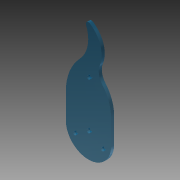
# Autodesk Inventor part: tail_bottom
Saved by Autodesk Inventor 2015 SP2 (Build 190223200, 223)
## iProperties
Created: 2015-10-08
Part Number: tail_bottom
Material: Generic
Document SubType Name: Modeling
Designer: styku
Density: 1 g/cm^3
Appearance: Clear
Author: styku
Autodesk Inventor part; units mm, degrees
ref_plane "YZ Plane" through (0, 0, 0) normal (1, 0, 0) x (0, 1, 0)
ref_plane "XZ Plane" through (0, 0, 0) normal (0, 1, 0) x (-1, 0, 0)
ref_plane "XY Plane" through (0, 0, 0) normal (0, 0, 1) x (1, 0, 0)
sketch "Sketch1" plane through (0, 0, 0) normal (0, 1, 0) x (-1, 0, 0)
  line L0 (46, 0) -> (-35, 0) construction
  line L1 (0, 54.3949) -> (0, -60) construction
  line L2 (22, -12.5) -> (22, 12.5)
  circle A0 centre (13.5, -18.75) radius 1.5
  line L3 (-22, 12.5) -> (-22, -12.5)
  circle A1 centre (0, 35) radius 1.5
  circle A2 centre (-13.5, -18.75) radius 1.5
  arc A3 (-22, -12.5) -> (22, -12.5) centre (0, -12) ccw
  arc A4 (-13.5294, 35.6977) -> (-11.0832, 50.96) centre (-25, 45.3634) ccw
  arc A5 (-13.5294, 35.6977) -> (-22, 12.5) centre (14, 12.5) ccw
  arc A6 (2.3262, 78.3342) -> (-1.3457, 81.3569) centre (0, 79.25) ccw
  arc A7 (-1.3457, 81.3569) -> (-11.0832, 50.96) centre (12.1114, 60.2879) ccw
  arc A8 (2.3262, 78.3342) -> (8.4007, 46.7782) centre (30.2411, 67.345) ccw
  arc A9 (22, 12.5) -> (8.4007, 46.7782) centre (-28, 12.5) ccw
  arc A10 (22, 12.5) -> (22, 12.5) centre (42.4714, 12.5) ccw
  circle A11 centre (0, -10) radius 1.75
  point P0 (0, 0)
  dimension "d16" = 3
  dimension "d44" = 3
  dimension "d53" = 12
  dimension "d54" = 25
  dimension "d56" = 5
  dimension "d57" = 15
  dimension "d58" = 36
  dimension "d59" = 50
  dimension "d60" = 25
  dimension "d61" = 30
  dimension "d62" = 0
  dimension "d64" = 25
  dimension "d67" = 44
  dimension "d68" = 35
  dimension "d69" = 18.75
  dimension "d70" = 27
  dimension "d71" = 12.1114
  dimension "d72" = 3.5
  dimension "d73" = 10
  constraints: 17 point on circle, 12 centre point, 9 tangent, 8 end point, 4 vertical, 3 point on line, 2 horizontal, 2 symmetric about line, 1 parallel, 2 other
  measures "d16" diameter of A0
  measures "d44" diameter of A1
  measures "d53" distance from line of L0 A3.centre
  measures "d54" distance of L3.start L3.end
  measures "d56" diameter of A6
  measures "d57" radius of A4
  measures "d58" radius of A5
  measures "d59" radius of A9
  measures "d60" radius of A7
  measures "d61" radius of A8
  measures "d62" distance from line of L1 A6.centre
  measures "d64" distance from line of L1 A4.centre
  measures "d67" distance between parallel lines of L3 L2
  measures "d68" distance from line of L0 A1.centre
  measures "d69" distance from line of L0 A2.centre
  measures "d70" distance of A2.centre A0.centre
  measures "d71" distance from line of L1 A7.centre
  measures "d72" diameter of A11
  measures "d73" distance from line of A11.centre L0
extrude "Extrusion4" add sketch "Sketch1" along normal blind 3 contours A3 L3 A5 A4 A7 A6 A8 A9 L2
body "Solid4"
